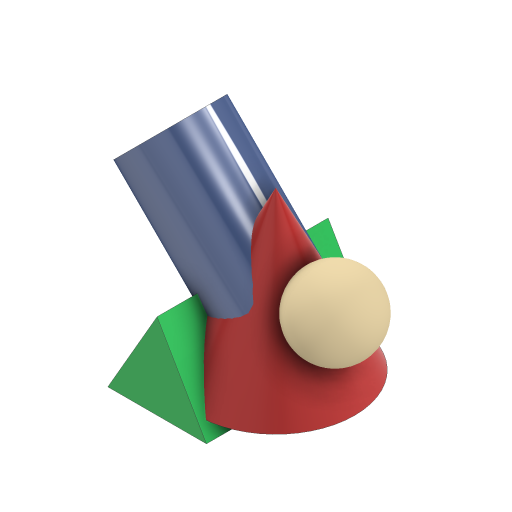
# Autodesk Inventor part: Лаба3
Saved by Autodesk Inventor 2023.2 (Build 272271030, 271C)
## iProperties
Created: 2023-09-30
Part Number: Лаба3
Material: Типовые
Document SubType Name: Modeling
Designer: User
Density: 1 g/cm^3
Appearance: По умолчанию
Author: User
Autodesk Inventor part; units mm, degrees
ref_plane "YZ Plane" through (0, 0, 0) normal (1, 0, 0) x (0, 1, 0)
ref_plane "XZ Plane" through (0, 0, 0) normal (0, 1, 0) x (-1, 0, 0)
ref_plane "XY Plane" through (0, 0, 0) normal (0, 0, 1) x (1, 0, 0)
sketch "Эскиз1" plane through (0, 0, 0) normal (0, 0, 1) x (1, 0, 0)
  line L0 (0, 0) -> (60, 0)
  line L1 (60, 0) -> (0, 120)
  line L2 (0, 120) -> (0, 0)
  dimension "d0" = 60
  dimension "d1" = 120
  constraints: 6 end point, 1 horizontal, 1 perpendicular
  measures "d0" distance of L0.start L0.end
  measures "d1" distance of L1.end L0.start
revolve "Вращение1" add sketch "Эскиз1" angle 360 about axis through (0, 120, 0) along (0, -1, 0)
sketch "Эскиз2" plane through (0, 0, 0) normal (0, 0, 1) x (1, 0, 0)
  line L0 (-60, 0) -> (60, 0) projected
  line L1 (0, 120) -> (60, 0) projected
  line L2 (45, 90) -> (45, 30)
  arc A0 (45, 30) -> (45, 90) centre (45, 60) ccw
  point P0 (0, 0)
  constraints: 2 end point, 2 point on circle, 1 centre point, 1 point on line
revolve "Вращение2" add sketch "Эскиз2" angle 360 about axis through (45, 90, 0) along (0, -1, 0) separate body
sketch "Эскиз5" plane through (0, 0, 0) normal (0, 0, 1) x (1, 0, 0)
  line L0 (-25.1641, 54.9519) -> (12.3359, -10)
  line L1 (12.3359, -10) -> (-62.6641, -10)
  line L2 (-62.6641, -10) -> (-25.1641, 54.9519)
  line L3 (-60, 0) -> (60, 0) projected
  point P0 (0, 0)
  dimension "d10" = 75
  dimension "d11" = 60
  dimension "d12" = 60
  dimension "d19" = 10
  constraints: 6 end point, 1 horizontal
  measures "d10" distance of L0.end L1.end
  measures "d11" angle of L1 L0
  measures "d12" angle of L1 L2
  measures "d19" distance from line of L3 L0.end
extrude "Выдавливание1" add sketch "Эскиз5" along normal mid plane 130 separate body
sketch "Эскиз6" plane through (0, 0, 0) normal (0, 0, 1) x (1, 0, 0)
  line L0 (0, 0) -> (0, 40)
  line L1 (0, 40) -> (-80, 120)
  line L2 (-80, 120) -> (-55, 145)
  line L3 (-55, 145) -> (25, 65)
  line L4 (25, 65) -> (0, 40)
  dimension "d22" = 40
  dimension "d23" = 25
  dimension "d25" = 80
  dimension "d26" = 135
  constraints: 10 end point, 3 perpendicular, 1 vertical
  measures "d22" distance of L0.start L0.end
  measures "d23" horizontal distance of L1.end L2.end
  measures "d25" horizontal distance of L3.end L2.end
  measures "d26" angle of L0 L1
revolve "Вращение3" add sketch "Эскиз6" angle 360 about axis through (0, 40, 0) along (-0.7071068, 0.7071068, 0) separate body
